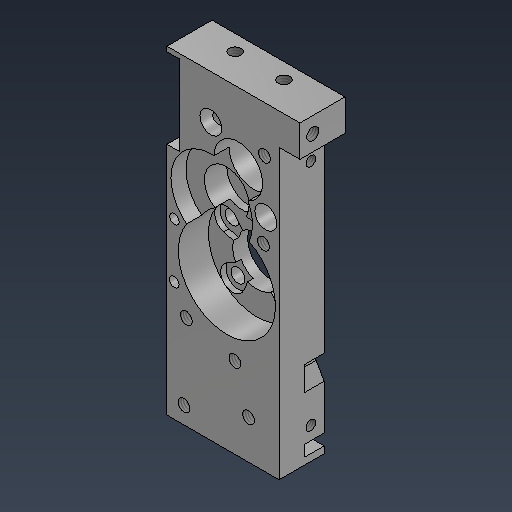
# Autodesk Inventor part: RightGearbox
Saved by Autodesk Inventor 2026.2 (Build 302298010, 298A)
## iProperties
Created: 2026-04-14
Part Number: RightGearbox
Material: Steel
Document SubType Name: Sheet Metal
Designer: szymo
Density: 7.85 g/cm^3
Appearance: Nylon 6(1)
Mass: 69.272 g
Surface Area: 68.2976 cm^2
Volume: 8.82446 cm^3
Sheet Metal Rule: Default
Author: szymo
Autodesk Inventor part; units mm, degrees
(part 1 of 2)
ref_plane "YZ Plane" through (0, 0, 0) normal (1, 0, 0) x (0, 1, 0)
ref_plane "XZ Plane" through (0, 0, 0) normal (0, 1, 0) x (-1, 0, 0)
ref_plane "XY Plane" through (0, 0, 0) normal (0, 0, 1) x (1, 0, 0)
sketch "Sketch1" plane through (0, 0, 0) normal (0, 0, 1) x (1, 0, 0)
  circle A0 centre (14.7, -14.7) radius 5
  circle A1 centre (14.7, -14.7) radius 14.7 construction
  circle A2 centre (14.7, -55.637072) radius 5
  circle A3 centre (14.7, -55.637072) radius 14.7 construction
  line L0 (23.1, 0) -> (0, 0)
  line L1 (0, 0) -> (0, -65.837072)
  line L2 (0, -65.837072) -> (23.1, -65.837072)
  line L3 (23.1, -65.837072) -> (23.1, 0)
  circle A4 centre (12.35, -35.272213) radius 5
  line L4 (23.43749, -53.479232) -> (27.439125, -51.168886)
  arc A5 (27.439125, -51.168886) -> (24.939125, -46.838759) centre (14.7, -55.637072) ccw
  line L5 (24.939125, -46.838759) -> (20.93749, -49.149105)
  arc A6 (23.43749, -53.479232) -> (20.93749, -49.149105) centre (14.7, -55.637072) ccw construction
  arc A7 (1.960875, -60.105258) -> (4.460875, -64.435385) centre (14.7, -55.637072) ccw
  line L6 (1.960875, -60.105258) -> (5.96251, -57.794913)
  line L7 (8.46251, -62.12504) -> (4.460875, -64.435385)
  line L8 (23.43749, -53.479232) -> (23.1, -53.479232)
  line L9 (24.939125, -46.838759) -> (23.1, -46.838759)
  line L10 (8.46251, -62.12504) -> (5.96251, -57.794913)
  line L11 (23.43749, -53.479232) -> (20.93749, -49.149105)
  line L12 (8.46251, -62.12504) -> (23.1, -62.12504)
  circle A8 centre (9.222618, -23.066498) radius 4.2 construction
  circle A9 centre (9.222618, -23.066498) radius 8 construction
  circle A10 centre (12.35, -35.272213) radius 9.6 construction
  circle A11 centre (12.35, -35.272213) radius 10
  circle A12 centre (9.222618, -23.066498) radius 4.6
  circle A13 centre (9.222618, -23.066498) radius 8.4
  arc A14 (5.96251, -57.794913) -> (8.46251, -62.12504) centre (14.7, -55.637072) ccw construction
  line L13 (2.5, -1) -> (1.5, -1)
  line L14 (1.5, -1) -> (1.5, -17)
  line L15 (1.5, -17) -> (2.5, -17)
  line L16 (2.5, -17) -> (2.5, -1)
  line L17 (1.5, -1) -> (1, -1)
  line L18 (1, -1) -> (1, -1)
  line L19 (1, -1) -> (0, -1)
  line L20 (2.5, -17) -> (2.5, -17.5)
  line L21 (2.5, -17.5) -> (1, -17.5)
  line L22 (1, -17.5) -> (1, -17.5)
  line L23 (1, -17.5) -> (0, -17.5)
  line L24 (23.1, 0) -> (27.4, 0)
  line L25 (27.4, 0) -> (27.4, -6.5)
  line L26 (27.4, -6.5) -> (23.1, -6.5)
  line L27 (24.939125, -23.498313) -> (20.93749, -21.187968)
  arc A15 (20.93749, -21.187968) -> (23.43749, -16.857841) centre (14.7, -14.7) ccw
  line L28 (23.43749, -16.857841) -> (27.439125, -19.168186)
  arc A16 (24.939125, -23.498313) -> (27.439125, -19.168186) centre (14.7, -14.7) ccw
  circle A17 centre (14.7, -14.7) radius 14.7 construction
  circle A18 centre (14.7, -14.7) radius 14 construction
  circle A19 centre (14.7, -14.7) radius 5
  circle A20 centre (14.7, -14.7) radius 14 construction
  line L29 (22.512272, -20.942468) -> (24.697093, -22.203875) construction
  arc A21 (22.512272, -20.942468) -> (24.012272, -18.344392) centre (14.7, -14.7) ccw construction
  line L30 (26.197093, -19.605799) -> (24.012272, -18.344392) construction
  arc A22 (24.697093, -22.203875) -> (26.197093, -19.605799) centre (14.7, -14.7) ccw construction
  circle A23 centre (14.7, -55.637072) radius 14.7 construction
  circle A24 centre (14.7, -55.637072) radius 14 construction
  line L31 (22.512272, -49.394604) -> (24.697093, -48.133197)
  arc A25 (26.197093, -50.731273) -> (24.697093, -48.133197) centre (14.7, -55.637072) ccw
  line L32 (26.197093, -50.731273) -> (24.012272, -51.99268)
  arc A26 (24.012272, -51.99268) -> (22.512272, -49.394604) centre (14.7, -55.637072) ccw
  arc A27 (3.202907, -60.542871) -> (4.702907, -63.140947) centre (14.7, -55.637072) ccw
  line L33 (3.202907, -60.542871) -> (5.387728, -59.281464)
  arc A28 (5.387728, -59.281464) -> (6.887728, -61.87954) centre (14.7, -55.637072) ccw
  line L34 (6.887728, -61.87954) -> (4.702907, -63.140947)
  circle A29 centre (14.7, -55.637072) radius 5
  circle A30 centre (14.7, -55.637072) radius 14 construction
  arc A31 (15.739868, -27.750823) -> (15.831115, -26.325602) centre (9.837244, -26.657388) ccw
  arc A32 (15.831115, -26.325602) -> (15.358114, -26.155676) centre (12.35, -35.272213) ccw
  arc A33 (15.358114, -26.155676) -> (14.521528, -27.313132) centre (19.770536, -30.225947) ccw
  arc A34 (14.521528, -27.313132) -> (14.102006, -27.210391) centre (12.35, -35.272213) ccw
  arc A35 (14.102006, -27.210391) -> (13.894939, -25.797343) centre (8.101031, -27.368074) ccw
  arc A36 (13.894939, -25.797343) -> (13.396945, -25.729472) centre (12.35, -35.272213) ccw
  arc A37 (13.396945, -25.729472) -> (12.819289, -27.035571) centre (18.559202, -28.793404) ccw
  arc A38 (12.819289, -27.035571) -> (12.387574, -27.022298) centre (12.35, -35.272213) ccw
  arc A39 (12.387574, -27.022298) -> (11.891242, -25.68318) centre (6.550518, -28.424209) ccw
  arc A40 (11.891242, -25.68318) -> (11.39002, -25.720331) centre (12.35, -35.272213) ccw
  arc A41 (11.39002, -25.720331) -> (11.09654, -27.117991) centre (17.076495, -27.644016) ccw
  arc A42 (11.09654, -27.117991) -> (10.671499, -27.194767) centre (12.35, -35.272213) ccw
  arc A43 (10.671499, -27.194767) -> (9.907595, -25.988105) centre (5.253471, -29.779634) ccw
  arc A44 (9.907595, -25.988105) -> (9.42505, -26.128654) centre (12.35, -35.272213) ccw
  arc A45 (9.42505, -26.128654) -> (9.428573, -27.556789) centre (15.387219, -26.828017) ccw
  arc A46 (9.428573, -27.556789) -> (9.028783, -27.720258) centre (12.35, -35.272213) ccw
  arc A47 (9.028783, -27.720258) -> (8.030693, -26.698789) centre (4.266575, -31.375112) ccw
  arc A48 (8.030693, -26.698789) -> (7.587914, -26.936594) centre (12.35, -35.272213) ccw
  arc A49 (7.587914, -26.936594) -> (7.888286, -28.332788) centre (13.565201, -26.381069) ccw
  arc A50 (7.888286, -28.332788) -> (7.53122, -28.575807) centre (12.35, -35.272213) ccw
  arc A51 (7.53122, -28.575807) -> (6.342565, -27.784174) centre (3.632965, -33.140911) ccw
  arc A52 (6.342565, -27.784174) -> (5.958905, -28.108841) centre (12.35, -35.272213) ccw
  arc A53 (5.958905, -28.108841) -> (6.542998, -29.412074) centre (11.690074, -26.322707) ccw
  arc A54 (6.542998, -29.412074) -> (6.24426, -29.72402) centre (12.35, -35.272213) ccw
  arc A55 (6.24426, -29.72402) -> (4.916991, -29.196821) centre (3.380331, -34.999859) ccw
  arc A56 (4.916991, -29.196821) -> (4.609216, -29.594161) centre (12.35, -35.272213) ccw
  arc A57 (4.609216, -29.594161) -> (5.451504, -30.747475) centre (9.843788, -26.655482) ccw
  arc A58 (5.451504, -30.747475) -> (5.224151, -31.114716) centre (12.35, -35.272213) ccw
  arc A59 (5.224151, -31.114716) -> (3.816275, -30.874993) centre (3.519714, -36.87071) ccw
  arc A60 (3.816275, -30.874993) -> (3.597838, -31.327639) centre (12.35, -35.272213) ccw
  arc A61 (3.597838, -31.327639) -> (4.661507, -32.28063) centre (8.107035, -27.364849) ccw
  arc A62 (4.661507, -32.28063) -> (4.515476, -32.687114) centre (12.35, -35.272213) ccw
  arc A63 (4.515476, -32.687114) -> (3.088524, -32.745344) centre (4.045023, -38.671698) ccw
  arc A64 (3.088524, -32.745344) -> (2.968971, -33.233515) centre (12.35, -35.272213) ccw
  arc A65 (2.968971, -33.233515) -> (4.207533, -33.944531) centre (6.555721, -28.419806) ccw
  arc A66 (4.207533, -33.944531) -> (4.149207, -34.372494) centre (12.35, -35.272213) ccw
  arc A67 (4.149207, -34.372494) -> (2.765544, -34.726131) centre (4.933299, -40.324113) ccw
  arc A68 (2.765544, -34.726131) -> (2.7501, -35.228491) centre (12.35, -35.272213) ccw
  arc A69 (2.7501, -35.228491) -> (4.109425, -35.666458) centre (5.257644, -29.774246) ccw
  arc A70 (4.109425, -35.666458) -> (4.141352, -36.097196) centre (12.35, -35.272213) ccw
  arc A71 (4.141352, -36.097196) -> (2.861451, -36.730784) centre (6.145721, -41.755736) ccw
  arc A72 (2.861451, -36.730784) -> (2.95079, -37.225378) centre (12.35, -35.272213) ccw
  arc A73 (2.95079, -37.225378) -> (4.37147, -37.371154) centre (4.269538, -31.368973) ccw
  arc A74 (4.37147, -37.371154) -> (4.492254, -37.785842) centre (12.35, -35.272213) ccw
  arc A75 (4.492254, -37.785842) -> (3.372052, -38.671691) centre (7.6293, -42.903997) ccw
  arc A76 (3.372052, -38.671691) -> (3.562271, -39.136902) centre (12.35, -35.272213) ccw
  arc A77 (3.562271, -39.136902) -> (4.982214, -38.984117) centre (3.634586, -33.134291) ccw
  arc A78 (4.982214, -38.984117) -> (5.186578, -39.36463) centre (12.35, -35.272213) ccw
  arc A79 (5.186578, -39.36463) -> (4.275033, -40.464025) centre (9.319196, -43.718713) ccw
  arc A80 (4.275033, -40.464025) -> (4.557818, -40.879521) centre (12.35, -35.272213) ccw
  arc A81 (4.557818, -40.879521) -> (5.914967, -40.434852) centre (3.38054, -34.993046) ccw
  arc A82 (5.914967, -40.434852) -> (6.193977, -40.76456) centre (12.35, -35.272213) ccw
  arc A83 (6.193977, -40.76456) -> (5.530929, -42.029451) centre (11.141552, -44.164277) ccw
  arc A84 (5.530929, -42.029451) -> (5.893921, -42.377073) centre (12.35, -35.272213) ccw
  arc A85 (5.893921, -42.377073) -> (7.128961, -41.659955) centre (3.518502, -36.864002) ccw
  arc A86 (7.128961, -41.659955) -> (7.470424, -41.924449) centre (12.35, -35.272213) ccw
  arc A87 (7.470424, -41.924449) -> (7.084851, -43.299554) centre (13.016724, -44.221214) ccw
  arc A88 (7.084851, -43.299554) -> (7.512186, -43.564109) centre (12.35, -35.272213) ccw
  arc A89 (7.512186, -43.564109) -> (8.571139, -42.605882) centre (4.042443, -38.665389) ccw
  arc A90 (8.571139, -42.605882) -> (8.960132, -42.793602) centre (12.35, -35.272213) ccw
  arc A91 (8.960132, -42.793602) -> (8.868885, -44.218823) centre (14.862756, -43.887037) ccw
  arc A92 (8.868885, -44.218823) -> (9.341886, -44.38875) centre (12.35, -35.272213) ccw
  arc A93 (9.341886, -44.38875) -> (10.178472, -43.231293) centre (4.929464, -40.318478) ccw
  arc A94 (10.178472, -43.231293) -> (10.597994, -43.334035) centre (12.35, -35.272213) ccw
  arc A95 (10.597994, -43.334035) -> (10.805061, -44.747083) centre (16.598969, -43.176351) ccw
  arc A96 (10.805061, -44.747083) -> (11.303055, -44.814954) centre (12.35, -35.272213) ccw
  arc A97 (11.303055, -44.814954) -> (11.880711, -43.508854) centre (6.140798, -41.751022) ccw
  arc A98 (11.880711, -43.508854) -> (12.312426, -43.522127) centre (12.35, -35.272213) ccw
  arc A99 (12.312426, -43.522127) -> (12.808758, -44.861245) centre (18.149482, -42.120216) ccw
  arc A100 (12.808758, -44.861245) -> (13.30998, -44.824094) centre (12.35, -35.272213) ccw
  arc A101 (13.30998, -44.824094) -> (13.60346, -43.426435) centre (7.623505, -42.90041) ccw
  arc A102 (13.60346, -43.426435) -> (14.028501, -43.349659) centre (12.35, -35.272213) ccw
  arc A103 (14.028501, -43.349659) -> (14.792405, -44.556321) centre (19.446529, -40.764791) ccw
  arc A104 (14.792405, -44.556321) -> (15.27495, -44.415771) centre (12.35, -35.272213) ccw
  arc A105 (15.27495, -44.415771) -> (15.271427, -42.987636) centre (9.312781, -43.716409) ccw
  arc A106 (15.271427, -42.987636) -> (15.671217, -42.824167) centre (12.35, -35.272213) ccw
  arc A107 (15.671217, -42.824167) -> (16.669307, -43.845636) centre (20.433425, -39.169314) ccw
  arc A108 (16.669307, -43.845636) -> (17.112086, -43.607831) centre (12.35, -35.272213) ccw
  arc A109 (17.112086, -43.607831) -> (16.811714, -42.211637) centre (11.134799, -44.163356) ccw
  arc A110 (16.811714, -42.211637) -> (17.16878, -41.968619) centre (12.35, -35.272213) ccw
  arc A111 (17.16878, -41.968619) -> (18.357435, -42.760252) centre (21.067035, -37.403514) ccw
  arc A112 (18.357435, -42.760252) -> (18.741095, -42.435585) centre (12.35, -35.272213) ccw
  arc A113 (18.741095, -42.435585) -> (18.157002, -41.132352) centre (13.009926, -44.221718) ccw
  arc A114 (18.157002, -41.132352) -> (18.45574, -40.820406) centre (12.35, -35.272213) ccw
  arc A115 (18.45574, -40.820406) -> (19.783009, -41.347604) centre (21.319669, -35.544567) ccw
  arc A116 (19.783009, -41.347604) -> (20.090784, -40.950264) centre (12.35, -35.272213) ccw
  arc A117 (20.090784, -40.950264) -> (19.248496, -39.79695) centre (14.856212, -43.888943) ccw
  arc A118 (19.248496, -39.79695) -> (19.475849, -39.42971) centre (12.35, -35.272213) ccw
  arc A119 (19.475849, -39.42971) -> (20.883725, -39.669433) centre (21.180286, -33.673716) ccw
  arc A120 (20.883725, -39.669433) -> (21.102162, -39.216786) centre (12.35, -35.272213) ccw
  arc A121 (21.102162, -39.216786) -> (20.038493, -38.263796) centre (16.592965, -43.179576) ccw
  arc A122 (20.038493, -38.263796) -> (20.184524, -37.857311) centre (12.35, -35.272213) ccw
  arc A123 (20.184524, -37.857311) -> (21.611476, -37.799082) centre (20.654977, -31.872727) ccw
  arc A124 (21.611476, -37.799082) -> (21.731029, -37.310911) centre (12.35, -35.272213) ccw
  arc A125 (21.731029, -37.310911) -> (20.492467, -36.599895) centre (18.144279, -42.12462) ccw
  arc A126 (20.492467, -36.599895) -> (20.550793, -36.171931) centre (12.35, -35.272213) ccw
  arc A127 (20.550793, -36.171931) -> (21.934456, -35.818295) centre (19.766701, -30.220312) ccw
  arc A128 (21.934456, -35.818295) -> (21.9499, -35.315935) centre (12.35, -35.272213) ccw
  arc A129 (21.9499, -35.315935) -> (20.590575, -34.877968) centre (19.442356, -40.77018) ccw
  arc A130 (20.590575, -34.877968) -> (20.558648, -34.44723) centre (12.35, -35.272213) ccw
  arc A131 (20.558648, -34.44723) -> (21.838549, -33.813641) centre (18.554279, -28.78869) ccw
  arc A132 (21.838549, -33.813641) -> (21.74921, -33.319048) centre (12.35, -35.272213) ccw
  arc A133 (21.74921, -33.319048) -> (20.32853, -33.173271) centre (20.430462, -39.175452) ccw
  arc A134 (20.32853, -33.173271) -> (20.207746, -32.758583) centre (12.35, -35.272213) ccw
  arc A135 (20.207746, -32.758583) -> (21.327948, -31.872734) centre (17.0707, -27.640428) ccw
  arc A136 (21.327948, -31.872734) -> (21.137729, -31.407523) centre (12.35, -35.272213) ccw
  arc A137 (21.137729, -31.407523) -> (19.717786, -31.560308) centre (21.065414, -37.410135) ccw
  arc A138 (19.717786, -31.560308) -> (19.513422, -31.179795) centre (12.35, -35.272213) ccw
  arc A139 (19.513422, -31.179795) -> (20.424967, -30.0804) centre (15.380804, -26.825712) ccw
  arc A140 (20.424967, -30.0804) -> (20.142182, -29.664905) centre (12.35, -35.272213) ccw
  arc A141 (20.142182, -29.664905) -> (18.785033, -30.109573) centre (21.31946, -35.551379) ccw
  arc A142 (18.785033, -30.109573) -> (18.506023, -29.779865) centre (12.35, -35.272213) ccw
  arc A143 (18.506023, -29.779865) -> (19.169071, -28.514974) centre (13.558448, -26.380149) ccw
  arc A144 (19.169071, -28.514974) -> (18.806079, -28.167352) centre (12.35, -35.272213) ccw
  arc A145 (18.806079, -28.167352) -> (17.571039, -28.884471) centre (21.181498, -33.680423) ccw
  arc A146 (17.571039, -28.884471) -> (17.229576, -28.619977) centre (12.35, -35.272213) ccw
  arc A147 (17.229576, -28.619977) -> (17.615149, -27.244871) centre (11.683276, -26.323211) ccw
  arc A148 (17.615149, -27.244871) -> (17.187814, -26.980316) centre (12.35, -35.272213) ccw
  arc A149 (17.187814, -26.980316) -> (16.128861, -27.938543) centre (20.657557, -31.879036) ccw
  arc A150 (16.128861, -27.938543) -> (15.739868, -27.750823) centre (12.35, -35.272213) ccw
  circle A151 centre (9.222618, -23.066498) radius 1.25
  arc A152 (17.179131, -22.233496) -> (16.013411, -21.993764) centre (15.595735, -26.978836) ccw
  arc A153 (16.013411, -21.993764) -> (15.947961, -21.639831) centre (9.222618, -23.066498) ccw
  arc A154 (15.947961, -21.639831) -> (16.950863, -20.999079) centre (13.775191, -17.133784) ccw
  arc A155 (16.950863, -20.999079) -> (16.832072, -20.597447) centre (9.222618, -23.066498) ccw
  arc A156 (16.832072, -20.597447) -> (15.641982, -20.605321) centre (16.269888, -25.568296) ccw
  arc A157 (15.641982, -20.605321) -> (15.504376, -20.27273) centre (9.222618, -23.066498) ccw
  arc A158 (15.504376, -20.27273) -> (16.352142, -19.437464) centre (12.442226, -16.316895) ccw
  arc A159 (16.352142, -19.437464) -> (16.152442, -19.069307) centre (9.222618, -23.066498) ccw
  arc A160 (16.152442, -19.069307) -> (14.989996, -19.324442) centre (16.636042, -24.048416) ccw
  arc A161 (14.989996, -19.324442) -> (14.786247, -19.027729) centre (9.222618, -23.066498) ccw
  arc A162 (14.786247, -19.027729) -> (15.441826, -18.034456) centre (10.968548, -15.794995) ccw
  arc A163 (15.441826, -18.034456) -> (15.169946, -17.715864) centre (9.222618, -23.066498) ccw
  arc A164 (15.169946, -17.715864) -> (14.085947, -18.20711) centre (16.678193, -22.485621) ccw
  arc A165 (14.085947, -18.20711) -> (13.824962, -17.959243) centre (9.222618, -23.066498) ccw
  arc A166 (13.824962, -17.959243) -> (14.259701, -16.851372) centre (9.418565, -15.590896) ccw
  arc A167 (14.259701, -16.851372) -> (13.927523, -16.596269) centre (9.222618, -23.066498) ccw
  arc A168 (13.927523, -16.596269) -> (12.969348, -17.302156) centre (16.3945, -20.948214) ccw
  arc A169 (12.969348, -17.302156) -> (12.662531, -17.113967) centre (9.222618, -23.066498) ccw
  arc A170 (12.662531, -17.113967) -> (12.857431, -15.939919) centre (7.860018, -15.713516) ccw
  arc A171 (12.857431, -15.939919) -> (12.479474, -15.759454) centre (9.222618, -23.066498) ccw
  arc A172 (12.479474, -15.759454) -> (11.688999, -16.649132) centre (15.797361, -19.503385) ccw
  arc A173 (11.688999, -16.649132) -> (11.34976, -16.528846) centre (9.222618, -23.066498) ccw
  arc A174 (11.34976, -16.528846) -> (11.296303, -15.339931) centre (6.361023, -16.157496) ccw
  arc A175 (11.296303, -15.339931) -> (10.889084, -15.241992) centre (9.222618, -23.066498) ccw
  arc A176 (10.889084, -15.241992) -> (10.300858, -16.276577) centre (14.912874, -18.214282) ccw
  arc A177 (10.300858, -16.276577) -> (9.944023, -16.229452) centre (9.222618, -23.066498) ccw
  arc A178 (9.944023, -16.229452) -> (9.644544, -15.077632) centre (4.987094, -16.903434) ccw
  arc A179 (9.644544, -15.077632) -> (9.225861, -15.066498) centre (9.222618, -23.066498) ccw
  arc A180 (9.225861, -15.066498) -> (8.865592, -16.200774) centre (13.779696, -17.137243) ccw
  arc A181 (8.865592, -16.200774) -> (8.506757, -16.228869) centre (9.222618, -23.066498) ccw
  arc A182 (8.506757, -16.228869) -> (7.974346, -15.164484) centre (3.798277, -17.918726) ccw
  arc A183 (7.974346, -15.164484) -> (7.562497, -15.240643) centre (9.222618, -23.066498) ccw
  arc A184 (7.562497, -15.240643) -> (7.445929, -16.425037) centre (12.447352, -16.319342) ccw
  arc A185 (7.445929, -16.425037) -> (7.100777, -16.527123) centre (9.222618, -23.066498) ccw
  arc A186 (7.100777, -16.527123) -> (6.358702, -15.596692) centre (2.84653, -19.159001) ccw
  arc A187 (6.358702, -15.596692) -> (5.971688, -15.756815) centre (9.222618, -23.066498) ccw
  arc A188 (5.971688, -15.756815) -> (6.103917, -16.939563) centre (10.974071, -15.796324) ccw
  arc A189 (6.103917, -16.939563) -> (5.787532, -17.11118) centre (9.222618, -23.066498) ccw
  arc A190 (5.787532, -17.11118) -> (4.868226, -16.355367) centre (2.173449, -20.570052) ccw
  arc A191 (4.868226, -16.355367) -> (4.52296, -16.592456) centre (9.222618, -23.066498) ccw
  arc A192 (4.52296, -16.592456) -> (4.898207, -17.721865) centre (9.424243, -15.591047) ccw
  arc A193 (4.898207, -17.721865) -> (4.624417, -17.955512) centre (9.222618, -23.066498) ccw
  arc A194 (4.624417, -17.955512) -> (3.568057, -17.40735) centre (1.80845, -22.09021) ccw
  arc A195 (3.568057, -17.40735) -> (3.27963, -17.711043) centre (9.222618, -23.066498) ccw
  arc A196 (3.27963, -17.711043) -> (3.881494, -18.737754) centre (7.865604, -15.712483) ccw
  arc A197 (3.881494, -18.737754) -> (3.662265, -19.023219) centre (9.222618, -23.066498) ccw
  arc A198 (3.662265, -19.023219) -> (2.51502, -18.706665) centre (1.767486, -23.653037) ccw
  arc A199 (2.51502, -18.706665) -> (2.296037, -19.063689) centre (9.222618, -23.066498) ccw
  arc A200 (2.296037, -19.063689) -> (3.098214, -19.94283) centre (6.366272, -16.155325) ccw
  arc A201 (3.098214, -19.94283) -> (2.943127, -20.267637) centre (9.222618, -23.066498) ccw
  arc A202 (2.943127, -20.267637) -> (1.755137, -20.196526) centre (2.052347, -25.190229) ccw
  arc A203 (1.755137, -20.196526) -> (1.615169, -20.591277) centre (9.222618, -23.066498) ccw
  arc A204 (1.615169, -20.591277) -> (2.5826, -21.284424) centre (4.991776, -16.900218) ccw
  arc A205 (2.5826, -21.284424) -> (2.498433, -21.634378) centre (9.222618, -23.066498) ccw
  arc A206 (2.498433, -21.634378) -> (1.321619, -21.811818) centre (2.650583, -26.634603) ccw
  arc A207 (1.321619, -21.811818) -> (1.266782, -22.227044) centre (9.222618, -23.066498) ccw
  arc A208 (1.266782, -22.227044) -> (2.357186, -22.703904) centre (3.802189, -17.914608) ccw
  arc A209 (2.357186, -22.703904) -> (2.347618, -23.06371) centre (9.222618, -23.066498) ccw
  arc A210 (2.347618, -23.06371) -> (1.233412, -23.481946) centre (3.536048, -27.923034) ccw
  arc A211 (1.233412, -23.481946) -> (1.266104, -23.8995) centre (9.222618, -23.066498) ccw
  arc A212 (1.266104, -23.8995) -> (2.431825, -24.139231) centre (2.8495, -19.154159) ccw
  arc A213 (2.431825, -24.139231) -> (2.497274, -24.493164) centre (9.222618, -23.066498) ccw
  arc A214 (2.497274, -24.493164) -> (1.494372, -25.133917) centre (4.670044, -28.999212) ccw
  arc A215 (1.494372, -25.133917) -> (1.613164, -25.535549) centre (9.222618, -23.066498) ccw
  arc A216 (1.613164, -25.535549) -> (2.803254, -25.527675) centre (2.175347, -20.564699) ccw
  arc A217 (2.803254, -25.527675) -> (2.940859, -25.860265) centre (9.222618, -23.066498) ccw
  arc A218 (2.940859, -25.860265) -> (2.093094, -26.695531) centre (6.003009, -29.816101) ccw
  arc A219 (2.093094, -26.695531) -> (2.292793, -27.063688) centre (9.222618, -23.066498) ccw
  arc A220 (2.292793, -27.063688) -> (3.45524, -26.808553) centre (1.809194, -22.084579) ccw
  arc A221 (3.45524, -26.808553) -> (3.658988, -27.105266) centre (9.222618, -23.066498) ccw
  arc A222 (3.658988, -27.105266) -> (3.003409, -28.09854) centre (7.476687, -30.338) ccw
  arc A223 (3.003409, -28.09854) -> (3.275289, -28.417132) centre (9.222618, -23.066498) ccw
  arc A224 (3.275289, -28.417132) -> (4.359288, -27.925885) centre (1.767042, -23.647374) ccw
  arc A225 (4.359288, -27.925885) -> (4.620274, -28.173753) centre (9.222618, -23.066498) ccw
  arc A226 (4.620274, -28.173753) -> (4.185534, -29.281624) centre (9.02667, -30.5421) ccw
  arc A227 (4.185534, -29.281624) -> (4.517712, -29.536727) centre (9.222618, -23.066498) ccw
  arc A228 (4.517712, -29.536727) -> (5.475887, -28.830839) centre (2.050736, -25.184782) ccw
  arc A229 (5.475887, -28.830839) -> (5.782704, -29.019028) centre (9.222618, -23.066498) ccw
  arc A230 (5.782704, -29.019028) -> (5.587804, -30.193077) centre (10.585217, -30.419479) ccw
  arc A231 (5.587804, -30.193077) -> (5.965762, -30.373541) centre (9.222618, -23.066498) ccw
  arc A232 (5.965762, -30.373541) -> (6.756236, -29.483864) centre (2.647875, -26.62961) ccw
  arc A233 (6.756236, -29.483864) -> (7.095475, -29.604149) centre (9.222618, -23.066498) ccw
  arc A234 (7.095475, -29.604149) -> (7.148932, -30.793064) centre (12.084212, -29.975499) ccw
  arc A235 (7.148932, -30.793064) -> (7.556152, -30.891003) centre (9.222618, -23.066498) ccw
  arc A236 (7.556152, -30.891003) -> (8.144378, -29.856418) centre (3.532361, -27.918714) ccw
  arc A237 (8.144378, -29.856418) -> (8.501212, -29.903544) centre (9.222618, -23.066498) ccw
  arc A238 (8.501212, -29.903544) -> (8.800691, -31.055364) centre (13.458141, -29.229562) ccw
  arc A239 (8.800691, -31.055364) -> (9.219374, -31.066497) centre (9.222618, -23.066498) ccw
  arc A240 (9.219374, -31.066497) -> (9.579644, -29.932221) centre (4.665539, -28.995752) ccw
  arc A241 (9.579644, -29.932221) -> (9.938479, -29.904126) centre (9.222618, -23.066498) ccw
  arc A242 (9.938479, -29.904126) -> (10.47089, -30.968511) centre (14.646958, -28.214269) ccw
  arc A243 (10.47089, -30.968511) -> (10.882738, -30.892352) centre (9.222618, -23.066498) ccw
  arc A244 (10.882738, -30.892352) -> (10.999306, -29.707959) centre (5.997884, -29.813653) ccw
  arc A245 (10.999306, -29.707959) -> (11.344458, -29.605872) centre (9.222618, -23.066498) ccw
  arc A246 (11.344458, -29.605872) -> (12.086533, -30.536303) centre (15.598705, -26.973994) ccw
  arc A247 (12.086533, -30.536303) -> (12.473547, -30.37618) centre (9.222618, -23.066498) ccw
  arc A248 (12.473547, -30.37618) -> (12.341319, -29.193432) centre (7.471164, -30.336672) ccw
  arc A249 (12.341319, -29.193432) -> (12.657703, -29.021816) centre (9.222618, -23.066498) ccw
  arc A250 (12.657703, -29.021816) -> (13.577009, -29.777628) centre (16.271786, -25.562943) ccw
  arc A251 (13.577009, -29.777628) -> (13.922275, -29.54054) centre (9.222618, -23.066498) ccw
  arc A252 (13.922275, -29.54054) -> (13.547029, -28.41113) centre (9.020992, -30.541949) ccw
  arc A253 (13.547029, -28.41113) -> (13.820819, -28.177483) centre (9.222618, -23.066498) ccw
  arc A254 (13.820819, -28.177483) -> (14.877178, -28.725645) centre (16.636785, -24.042785) ccw
  arc A255 (14.877178, -28.725645) -> (15.165605, -28.421953) centre (9.222618, -23.066498) ccw
  arc A256 (15.165605, -28.421953) -> (14.563742, -27.395241) centre (10.579632, -30.420512) ccw
  arc A257 (14.563742, -27.395241) -> (14.782971, -27.109776) centre (9.222618, -23.066498) ccw
  arc A258 (14.782971, -27.109776) -> (15.930215, -27.42633) centre (16.67775, -22.479959) ccw
  arc A259 (15.930215, -27.42633) -> (16.149199, -27.069306) centre (9.222618, -23.066498) ccw
  arc A260 (16.149199, -27.069306) -> (15.347022, -26.190166) centre (12.078963, -29.97767) ccw
  arc A261 (15.347022, -26.190166) -> (15.502108, -25.865358) centre (9.222618, -23.066498) ccw
  arc A262 (15.502108, -25.865358) -> (16.690098, -25.936469) centre (16.392889, -20.942767) ccw
  arc A263 (16.690098, -25.936469) -> (16.830067, -25.541718) centre (9.222618, -23.066498) ccw
  arc A264 (16.830067, -25.541718) -> (15.862636, -24.848571) centre (13.453459, -29.232777) ccw
  arc A265 (15.862636, -24.848571) -> (15.946802, -24.498617) centre (9.222618, -23.066498) ccw
  arc A266 (15.946802, -24.498617) -> (17.123616, -24.321177) centre (15.794653, -19.498392) ccw
  arc A267 (17.123616, -24.321177) -> (17.178453, -23.905951) centre (9.222618, -23.066498) ccw
  arc A268 (17.178453, -23.905951) -> (16.088049, -23.429091) centre (14.643046, -28.218388) ccw
  arc A269 (16.088049, -23.429091) -> (16.097617, -23.069285) centre (9.222618, -23.066498) ccw
  arc A270 (16.097617, -23.069285) -> (17.211823, -22.651049) centre (14.909187, -18.209961) ccw
  arc A271 (17.211823, -22.651049) -> (17.179131, -22.233496) centre (9.222618, -23.066498) ccw
  circle A272 centre (9.222618, -23.066498) radius 1.25
  arc A273 (5.454999, -24.922583) -> (6.852288, -24.648912) centre (5.454876, -21.21803) ccw
  arc A274 (6.852288, -24.648912) -> (7.079113, -24.944764) centre (9.222618, -23.066498) ccw
  arc A275 (7.079113, -24.944764) -> (6.452085, -26.223102) centre (10.029598, -27.184931) ccw
  arc A276 (6.452085, -26.223102) -> (6.887807, -26.557724) centre (9.222618, -23.066498) ccw
  arc A277 (6.887807, -26.557724) -> (7.961059, -25.622074) centre (5.035423, -23.349549) ccw
  arc A278 (7.961059, -25.622074) -> (8.305421, -25.764877) centre (9.222618, -23.066498) ccw
  arc A279 (8.305421, -25.764877) -> (8.401568, -27.185463) centre (11.9807, -26.229676) ccw
  arc A280 (8.401568, -27.185463) -> (8.946225, -27.257393) centre (9.222618, -23.066498) ccw
  arc A281 (8.946225, -27.257393) -> (9.407864, -25.910471) centre (5.737927, -25.405224) ccw
  arc A282 (9.407864, -25.910471) -> (9.777492, -25.861961) centre (9.222618, -23.066498) ccw
  arc A283 (9.777492, -25.861961) -> (10.571051, -27.044151) centre (13.192776, -24.42685) ccw
  arc A284 (10.571051, -27.044151) -> (11.078703, -26.834116) centre (9.222618, -23.066498) ccw
  arc A285 (11.078703, -26.834116) -> (10.805032, -25.436828) centre (7.37415, -26.83424) ccw
  arc A286 (10.805032, -25.436828) -> (11.100884, -25.210003) centre (9.222618, -23.066498) ccw
  arc A287 (11.100884, -25.210003) -> (12.379222, -25.83703) centre (13.341052, -22.259518) ccw
  arc A288 (12.379222, -25.83703) -> (12.713844, -25.401308) centre (9.222618, -23.066498) ccw
  arc A289 (12.713844, -25.401308) -> (11.778194, -24.328057) centre (9.505669, -27.253692) ccw
  arc A290 (11.778194, -24.328057) -> (11.920997, -23.983694) centre (9.222618, -23.066498) ccw
  arc A291 (11.920997, -23.983694) -> (13.341583, -23.887547) centre (12.385796, -20.308416) ccw
  arc A292 (13.341583, -23.887547) -> (13.413513, -23.34289) centre (9.222618, -23.066498) ccw
  arc A293 (13.413513, -23.34289) -> (12.066591, -22.881252) centre (11.561344, -26.551189) ccw
  arc A294 (12.066591, -22.881252) -> (12.018081, -22.511624) centre (9.222618, -23.066498) ccw
  arc A295 (12.018081, -22.511624) -> (13.200271, -21.718065) centre (10.58297, -19.096339) ccw
  arc A296 (13.200271, -21.718065) -> (12.990236, -21.210413) centre (9.222618, -23.066498) ccw
  arc A297 (12.990236, -21.210413) -> (11.592948, -21.484083) centre (12.99036, -24.914965) ccw
  arc A298 (11.592948, -21.484083) -> (11.366123, -21.188231) centre (9.222618, -23.066498) ccw
  arc A299 (11.366123, -21.188231) -> (11.99315, -19.909894) centre (8.415638, -18.948064) ccw
  arc A300 (11.99315, -19.909894) -> (11.557428, -19.575272) centre (9.222618, -23.066498) ccw
  arc A301 (11.557428, -19.575272) -> (10.484177, -20.510922) centre (13.409812, -22.783446) ccw
  arc A302 (10.484177, -20.510922) -> (10.139814, -20.368118) centre (9.222618, -23.066498) ccw
  arc A303 (10.139814, -20.368118) -> (10.043667, -18.947532) centre (6.464536, -19.903319) ccw
  arc A304 (10.043667, -18.947532) -> (9.49901, -18.875602) centre (9.222618, -23.066498) ccw
  arc A305 (9.49901, -18.875602) -> (9.037372, -20.222524) centre (12.707309, -20.727771) ccw
  arc A306 (9.037372, -20.222524) -> (8.667744, -20.271034) centre (9.222618, -23.066498) ccw
  arc A307 (8.667744, -20.271034) -> (7.874185, -19.088844) centre (5.252459, -21.706146) ccw
  arc A308 (7.874185, -19.088844) -> (7.366533, -19.298879) centre (9.222618, -23.066498) ccw
  arc A309 (7.366533, -19.298879) -> (7.640203, -20.696167) centre (11.071085, -19.298755) ccw
  arc A310 (7.640203, -20.696167) -> (7.344351, -20.922993) centre (9.222618, -23.066498) ccw
  arc A311 (7.344351, -20.922993) -> (6.066014, -20.295965) centre (5.104184, -23.873478) ccw
  arc A312 (6.066014, -20.295965) -> (5.731392, -20.731687) centre (9.222618, -23.066498) ccw
  arc A313 (5.731392, -20.731687) -> (6.667042, -21.804939) centre (8.939567, -18.879303) ccw
  arc A314 (6.667042, -21.804939) -> (6.524238, -22.149301) centre (9.222618, -23.066498) ccw
  arc A315 (6.524238, -22.149301) -> (5.103652, -22.245448) centre (6.059439, -25.82458) ccw
  arc A316 (5.103652, -22.245448) -> (5.031722, -22.790105) centre (9.222618, -23.066498) ccw
  arc A317 (5.031722, -22.790105) -> (6.378644, -23.251744) centre (6.883891, -19.581807) ccw
  arc A318 (6.378644, -23.251744) -> (6.427154, -23.621372) centre (9.222618, -23.066498) ccw
  arc A319 (6.427154, -23.621372) -> (5.244964, -24.414931) centre (7.862266, -27.036656) ccw
  arc A320 (5.244964, -24.414931) -> (5.454999, -24.922583) centre (9.222618, -23.066498) ccw
  line L35 (1.5, -17) -> (1.5, -1)
  line L36 (2.5, -17) -> (1.5, -17)
  line L37 (2.5, -1) -> (2.5, -17)
  line L38 (2.5, -1) -> (1.5, -1)
  line L39 (4.460875, -64.435385) -> (23.1, -64.435385)
  point P0 (0, 0)
  point P1 (4.394176, -65.837072)
  point P2 (4.054242, -29.688272)
  point P3 (9.70004, -14.680076)
  point P4 (16.718073, -19.274645)
  point P5 (16.938443, -26.387046)
  point P6 (6.782075, -26.965696)
  point P7 (13.237489, -25.311672)
  point P8 (10.057406, -65.837072)
  point P9 (23.1, -47.900579)
  point P10 (23.1, -52.894682)
  dimension "d2" = 4.5
  dimension "d3" = 6.3
  dimension "d4" = 0.4
  dimension "d5" = 0.4
  dimension "d6" = 0.4
  dimension "d27" = 0
  dimension "d36" = 0.5
  dimension "d37" = 0
  dimension "d38" = 0.5
  dimension "d39" = 0.5
  dimension "d40" = 0
  dimension "d41" = 2
  dimension "d43" = 10
  dimension "d44" = 1
  dimension "d45" = 1
  dimension "d46" = 1
  dimension "d47" = 1
  dimension "d48" = 1
  dimension "d49" = 1
  dimension "d50" = 1
  dimension "d51" = 1
  dimension "d52" = 1
  dimension "d54" = 1
  dimension "d56" = 1
  dimension "d57" = 1
  dimension "d112" = 6.5
  constraints: 60 end point, 14 centre point, 13 coincident, 13 perpendicular, 12 point on circle, 7 parallel, 7 point on line, 6 tangent, 4 horizontal, 1 collinear, 1 vertical, 13 other
  measures "d2" distance edge to line of A3 L2
  measures "d3" distance edge to line of A1 L3
  measures "d27" distance from line of L6 A14.start
  measures "d36" distance between parallel lines of L14 L18
  measures "d37" distance between parallel lines of L19 L13
  measures "d38" distance between parallel lines of L22 L14
  measures "d39" distance between parallel lines of L21 L15
  measures "d40" distance between parallel lines of L21 L23
  measures "d41" distance edge to line of A1 L25
  measures "d43" diameter of A4
  measures "d44" distance between parallel lines of L28 L30
  measures "d45" distance between parallel lines of L27 L29
  measures "d46" radial gap between concentric circles of A22 A16
  measures "d47" radial gap between concentric circles of A15 A21
  measures "d48" distance between parallel lines of L32 L4
  measures "d49" distance between parallel lines of L5 L31
  measures "d50" radial gap between concentric circles of A5 A25
  measures "d51" radial gap between concentric circles of A6 A26
  measures "d52" radial gap between concentric circles of A28 A14
  measures "d54" radial gap between concentric circles of A7 A27
  measures "d56" distance between parallel lines of L6 L33
  measures "d57" distance between parallel lines of L7 L34
  measures "d112" distance between parallel lines of L26 L24
extrude "Extrusion5" add sketch "Sketch1" along normal blind 3.1 contours A0 A178 A179 A180 A181 A182 A183 A184 A185 A186 A187 A188 A189 A190 A191 A192 A193 A194 A195 A196 A197 A198 A199 A200 A201 A202 A203 A204 A205 A206 A207 A208 A209 A210 A211 A212 A213 A214 A215 A216 A217 A218 A219 A220 A221 A222 A223 A224 A225 A226 A227 A11 A13 | A13 A11 A262 A263 A264 A265 A266 A267 A268 A269 A270 A271 A152 A153 A154 A155 A156 A157 A158 A159 A0 | A0 A159 A158 A157 A156 A155 A154 A153 A152 A271 A270 A269 A268 A267 A266 A265 A264 A263 A262 A11 A12 A227 A226 A225 A224 A223 A222 A221 A220 A219 A218 A217 A216 A215 A214 A213 A212 A211 A210 A209 A208 A207 A206 A205 A204 A203 A202 A201 A200 A199 A198 A197 A196 A195 A194 A193 A192 A191 A190 A189 A188 A187 A186 A185 A184 A183 A182 A181 A180 A179 A178 | A13 A57 A58 A59 A60 A61 A62 A63 A64 A65 A66 A67 A68 A69 A70 A71 A72 A73 A74 A75 A76 A77 A78 A79 A80 A81 A82 A83 A84 A85 A86 A87 A88 A89 A90 A91 A92 A93 A94 A95 A96 A97 A98 A99 A100 A101 A102 A103 A104 A105 A106 A107 A108 A109 A110 A111 A112 A113 A114 A115 A116 A117 A118 A119 A120 A121 A122 A123 A124 A125 A126 A127 A128 A129 A130 A131 A132 A133 A134 A135 A136 A137 A138 A139 A140 A141 A142 A143 A144 A145 A146 A147 A148 A149 A150 A11 | A11 A227 A228 A56 A57 A13 | A11 A12 A49 A50 A51 A52 A53 A54 A55 A230 A229 A228 A56 A227 | A57 A56 A228 A55 A230 A231 A232 A233 A234 A235 A236 A237 A238 A239 A240 A241 A242 A4 A13 | A13 A4 A150 A149 A148 A147 A146 A145 A144 A143 A142 A141 A140 A139 A138 A137 A136 A135 A134 A133 A132 A131 A130 A129 A128 A127 A126 A125 A124 A123 A122 A121 A120 A119 A118 A117 A116 A115 A114 A113 A112 A111 A110 A109 A108 A107 A106 A105 A104 A103 A102 A101 A100 A99 A98 A97 A96 A95 A94 A93 A92 A91 A90 A89 A88 A87 A86 A85 A84 A83 A82 A81 A80 A79 A78 A77 A76 A75 A74 A73 A72 A71 A70 A69 A68 A67 A66 A65 A64 A63 A62 A61 A60 A59 A58 A57 | A13 A150 A31 A258 A259 A260 A32 A261 A262 A11 | A262 A261 A32 A33 A34 A35 A36 A37 A38 A39 A12 A11 | A13 A4 A248 A249 A250 A251 A252 A253 A254 A255 A256 A257 A258 A31 A150 | A12 A47 A46 A39 A38 A37 A36 A35 A34 A33 A32 A261 A260 A31 A258 A257 A256 A255 A254 A253 A252 A251 A250 A249 A248 A4 A246 A245 A244 A242 A241 A240 A239 A238 A237 A236 A235 A234 A233 A232 A231 A230 A55 A54 A53 A52 A51 A50 A49 | A56 A55 A228 | A12 A46 A47 | A228 A229 A230 A55 | A244 A245 A246 A4 | A32 A31 A260 A261 | A31 A260 A259 A258 | A2 | L3 A15 L27 L5 L11 L12 L10 L6 A7 L39 L2 L1 L23 L21 L20 L16 L13 L17 L19 L0 | L24 L25 L26 L3 | L3 L27 A15 | L3 L31 A26 L11 L5 | L39 L7 L12 L3 | L3 A26 L31 | A7 L6 L10 L7 | L33 A28 L34 A27
extrude "Extrusion6" add sketch "Sketch1" along normal blind 6.2 contours A0 A178 A179 A180 A181 A182 A183 A184 A185 A186 A187 A188 A189 A190 A191 A192 A193 A194 A195 A196 A197 A198 A199 A200 A201 A202 A203 A204 A205 A206 A207 A208 A209 A210 A211 A212 A213 A214 A215 A216 A217 A218 A219 A220 A221 A222 A223 A224 A225 A226 A227 A11 A13 | A13 A11 A262 A263 A264 A265 A266 A267 A268 A269 A270 A271 A152 A153 A154 A155 A156 A157 A158 A159 A0 | A0 A159 A158 A157 A156 A155 A154 A153 A152 A271 A270 A269 A268 A267 A266 A265 A264 A263 A262 A11 A12 A227 A226 A225 A224 A223 A222 A221 A220 A219 A218 A217 A216 A215 A214 A213 A212 A211 A210 A209 A208 A207 A206 A205 A204 A203 A202 A201 A200 A199 A198 A197 A196 A195 A194 A193 A192 A191 A190 A189 A188 A187 A186 A185 A184 A183 A182 A181 A180 A179 A178 | A2 | L3 A15 L27 L5 L11 L12 L10 L6 A7 L39 L2 L1 L23 L21 L20 L16 L13 L17 L19 L0 | L24 L25 L26 L3 | L3 L27 A15 | L3 L31 A26 L11 L5 | L39 L7 L12 L3 | L3 A26 L31 | A7 L6 L10 L7 | L33 A28 L34 A27
ref_plane "Work Plane3" through (6.764102, -40.858111, 9.3) normal (0, 0, 1) x (0.9993859, -0.0350396, 0)
extrude "Extrusion7" add sketch "Sketch1" along normal up to surface (9.3 mm away) contours A2 | L3 A15 L27 L5 L11 L12 L10 L6 A7 L39 L2 L1 L23 L21 L20 L16 L13 L17 L19 L0 | L24 L25 L26 L3 | L3 L27 A15 | L3 L31 A26 L11 L5 | L39 L7 L12 L3 | L3 A26 L31 | A7 L6 L10 L7 | L33 A28 L34 A27
extrude "Extrusion8" cut sketch "Sketch1" along normal blind 4 contours A2 | L3 L31 A26 L11 L5 | L39 L7 L12 L3 | L3 A26 L31 | A7 L6 L10 L7 | L33 A28 L34 A27
sketch "Sketch3" plane through (0, -65.837072, 9.3) normal (0, -1, 0) x (1, 0, 0)
  line L0 (23.1, -9.3) -> (23.1, 0) projected
  line L1 (23.1, 0) -> (0, 0) projected
  line L2 (0, -9.3) -> (0, 0) projected
  circle A0 centre (13.55, -3) radius 3
  circle A1 centre (7, -3) radius 3
  line L3 (4, -9.3) -> (4, 0)
  line L4 (0, -9.3) -> (23.1, -9.3) projected
  circle A2 centre (20.1, -3) radius 3
  line L5 (23.1, -9.3) -> (23.1, 0) projected
  line L6 (23.1, 0) -> (0, 0) projected
  point P0 (0, -9.3)
  dimension "d71" = 6
  dimension "d72" = 6
  dimension "d73" = 4
  dimension "d188" = 6
  dimension "d189" = 6.55
  dimension "d190" = 6.55
  constraints: 5 tangent, 3 centre point, 2 end point, 1 perpendicular, 1 point on line
  measures "d71" diameter of A1
  measures "d72" diameter of A0
  measures "d73" distance between parallel lines of L2 L3
  measures "d188" diameter of A2
  measures "d189" distance of A0.centre A2.centre
  measures "d190" distance of A1.centre A0.centre
hole "Hole1" at (13.55, -65.837072, 6.3) at (7, -65.837072, 6.3) at (20.1, -65.837072, 6.3) direction (0, 1, 0) diameter 2.459 depth 10 thread size "M3x0.5" class "6H" standard "ISO Metric profile"
sketch "Sketch4" plane through (0, 0, 9.3) normal (0, 0, 1) x (1, 0, 0)
  arc A0 (4.054242, -29.688272) -> (16.938443, -26.387046) centre (12.35, -35.272213) ccw
  arc A1 (9.70004, -14.680076) -> (4.054242, -29.688272) centre (9.222618, -23.066498) ccw
  arc A2 (16.718073, -19.274645) -> (9.70004, -14.680076) centre (14.7, -14.7) ccw
  arc A3 (16.938443, -26.387046) -> (16.718073, -19.274645) centre (9.222618, -23.066498) ccw
  line L0 (27.4, 0) -> (27.4, -6.5)
  line L1 (0, 0) -> (27.4, 0)
  line L2 (0, -1) -> (0, 0)
  line L3 (2.5, -1) -> (0, -1)
  line L4 (2.5, -17.5) -> (2.5, -1)
  line L5 (0, -17.5) -> (2.5, -17.5)
  line L6 (0, -65.837072) -> (0, -17.5)
  line L7 (23.1, -6.5) -> (23.1, -65.837072)
  line L8 (27.4, -6.5) -> (23.1, -6.5)
  line L9 (23.1, -6.5) -> (2.5, -6.5)
  line L10 (23.1, -19.5) -> (2.5, -19.5)
  circle A4 centre (16.825, -57.837072) radius 3
  circle A5 centre (3.5, -62.337072) radius 3.5
  line L11 (0, -65.837072) -> (0, 0)
  line L12 (23.1, -65.837072) -> (0, -65.837072)
  line L13 (23.1, -6.5) -> (23.1, -65.837072)
  circle A6 centre (20.104628, -9.5) radius 3
  circle A7 centre (20.104628, -9.5) radius 2.5
  arc A8 (16.718073, -19.274645) -> (9.70004, -14.680076) centre (14.7, -14.7) ccw
  circle A9 centre (4, -46.509539) radius 4
  circle A10 centre (14, -49.174641) radius 4
  arc A11 (4.054242, -29.688272) -> (16.938443, -26.387046) centre (12.35, -35.272213) ccw
  circle A12 centre (19.890727, -25.302888) radius 3
  circle A13 centre (19.890727, -25.302888) radius 2.5
  line L14 (23.1, -65.837072) -> (0, -65.837072)
  line L15 (21.3295, -65.837072) -> (18.8705, -65.837072)
  line L16 (14.7795, -65.837072) -> (12.3205, -65.837072)
  line L17 (12.3205, -55.837072) -> (14.7795, -55.837072)
  line L18 (21.3295, -65.837072) -> (18.8705, -65.837072)
  line L19 (18.8705, -55.837072) -> (21.3295, -55.837072)
  point P0 (0, -15)
  dimension "d85" = 6.5
  dimension "d86" = 19.5
  dimension "d87" = 6
  dimension "d88" = 7
  dimension "d89" = 6
  dimension "d90" = 5
  dimension "d92" = 8
  dimension "d93" = 8
  dimension "d94" = 6
  dimension "d95" = 5
  dimension "d103" = 10
  dimension "d191" = 5
  dimension "d192" = 4.5045
  dimension "d193" = 4.5045
  constraints: 9 tangent, 8 centre point, 4 end point, 4 point on line, 2 coincident, 1 parallel, 1 perpendicular
  measures "d85" distance between parallel lines of L1 L9
  measures "d86" distance between parallel lines of L1 L10
  measures "d87" diameter of A4
  measures "d88" diameter of A5
  measures "d89" diameter of A6
  measures "d90" diameter of A7
  measures "d92" diameter of A9
  measures "d93" diameter of A10
  measures "d94" diameter of A12
  measures "d95" diameter of A13
  measures "d103" horizontal distance of A9.centre A10.centre
  measures "d191" distance edge to line of A4 L12
  measures "d192" horizontal distance of A4.centre L19.end
  measures "d193" horizontal distance of A4.centre L17.start
sketch "Sketch12" plane through (0, 0, 9.3) normal (0, 0, 1) x (1, 0, 0)
  circle A0 centre (20.356854, -20.356854) radius 1.05643
  circle A1 centre (9.043146, -9.043146) radius 1.05643
  circle A2 centre (14.7, -14.7) radius 5
  circle A3 centre (14.7, -14.7) radius 14
  point P0 (0, 0)
hole "Hole9" at (9.043146, -9.043146, 9.3) at (20.356854, -20.356854, 9.3) direction (0, 0, -1) diameter 2.5 depth 10.3 counterbore diameter 4.5 counterbore depth 5.3
hole "Hole2" at (14, -49.174641, 9.3) at (19.890727, -25.302888, 9.3) at (16.825, -57.837072, 9.3) at (3.5, -62.337072, 9.3) at (4, -46.509539, 9.3) at (20.104628, -9.5, 9.3) direction (0, 0, -1) diameter 2.459 depth 15.55 thread size "M3x0.5" class "6H" standard "ISO Metric profile"
sketch "Sketch6" plane through (27.4, -6.5, 0) normal (1, 0, 0) x (0, 0, -1)
  line L0 (0, 0) -> (0, 6.5) projected
  line L1 (0, 6.5) -> (-9.3, 6.5) projected
  line L2 (-9.3, 6.5) -> (-9.3, 0) projected
  line L3 (0, 0) -> (-9.3, 0) projected
  line L4 (-4, 0) -> (-4, 6.5)
  line L5 (0, 0) -> (-9.3, 0) projected
  line L6 (-4, 0) -> (-9.3, 6.5)
  line L7 (-9.3, 6.5) -> (-9.3, 0) projected
  line L8 (-4, 6.5) -> (-9.3, 0)
  point P0 (0, 6.5)
  point P1 (-6.65, 3.25)
  dimension "d217" = 5.3
  constraints: 6 end point, 2 midpoint, 2 point on line, 1 perpendicular
  measures "d217" distance between parallel lines of L2 L4
hole "Hole4" at (27.4, -3.25, 6.65) direction (-1, 0, 0) diameter 2.459 depth 10 thread size "M3x0.5" class "6H" standard "ISO Metric profile"
sketch "Sketch5" plane through (0, -65.837072, 0) normal (-1, 0, 0) x (0, 0, 1)
  line L0 (-3.8, 40.042024) -> (-3.8, 20.295048)
  line L1 (0, 40.042024) -> (0, 20.295048)
  line L2 (0, 40.042024) -> (-3.8, 40.042024)
  circle A0 centre (-1.9, 30.668536) radius 1.0065
  line L3 (0, 20.295048) -> (-3.8, 20.295048)
  point P0 (0, 65.837072)
hole "Hole3" at (0, -35.168536, -1.9) direction (1, 0, 0) diameter 2.9 end through all countersink diameter 7 countersink angle 90 clearance for "Countersunk Flat Head Screw ISO 2009/7046" size "M2.5" standard "ISO"
sketch "Sketch7" plane through (23.1, -65.837072, 9.3) normal (1, 0, 0) x (0, 0, -1)
  line L0 (5.3, 1.401687) -> (5.3, 3.712032)
  line L1 (9.3, 59.337072) -> (0, 59.337072)
  line L2 (0, 59.337072) -> (0, 0)
  line L3 (9.3, 0) -> (0, 0)
  circle A0 centre (6.55, 53.607572) radius 2.75
  line L4 (9.3, 59.337072) -> (0, 59.337072)
  circle A1 centre (6.55, 6.462032) radius 2.75
  line L5 (5.3, 17.936494) -> (9.3, 17.936494)
  line L6 (9.3, 17.936494) -> (9.3, 59.337072)
  line L7 (9.3, 0) -> (9.3, 1.401687)
  line L8 (9.3, 12.94239) -> (5.3, 12.94239)
  line L9 (9.3, 1.401687) -> (5.3, 1.401687)
  line L10 (5.3, 3.712032) -> (9.3, 3.712032)
  line L11 (9.3, 3.712032) -> (9.3, 12.94239)
  line L12 (5.3, 12.94239) -> (5.3, 17.936494)
  line L13 (9.3, 57.566572) -> (9.3, 55.107572)
  line L14 (0, 55.107572) -> (0, 57.566572)
  point P0 (9.3, 65.837072)
  dimension "d122" = 5.5
  dimension "d123" = 5.5
  dimension "d194" = 1.5
  constraints: 3 tangent, 2 centre point
  measures "d122" diameter of A0
  measures "d123" diameter of A1
  measures "d194" vertical distance of A0.centre L13.end
hole "Hole5" at (23.1, -59.37504, 2.75) at (23.1, -12.2295, 2.75) direction (-1, 0, 0) diameter 2.013 depth 8 thread size "M2.5x0.45" class "6H" standard "ISO Metric profile"